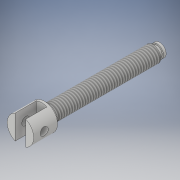
# Autodesk Inventor part: крепёж
Saved by Autodesk Inventor 2019 (Build 230136000, 136)
## iProperties
Created: 2019-04-29
Part Number: крепёж
Material: Типовые
Document SubType Name: Modeling
Designer: BarmanKaktus
Density: 1 g/cm^3
Appearance: По умолчанию
Author: BarmanKaktus
Autodesk Inventor part; units mm, degrees
sketch "Эскиз1" plane through (0, 0, 0) normal (0, 0, 1) x (1, 0, 0)
  circle A0 centre (0, 0) radius 3
  dimension "d0" = 6
  constraints: 1 centre point, 1 coincident
  measures "d0" diameter of A0
extrude "Выдавливание1" add sketch "Эскиз1" along normal blind 40
ref_plane "РабПлоскость1" through (0, 0, 40) normal (0, 0, 1) x (1, 0, 0)
sketch "Эскиз2" plane through (0, 0, 40) normal (0, 0, 1) x (1, 0, 0)
  circle A0 centre (0, 0) radius 5
  dimension "d4" = 10
  constraints: 1 centre point, 1 coincident
  measures "d4" diameter of A0
extrude "Выдавливание2" add sketch "Эскиз2" along normal blind 10
ref_plane "РабПлоскость2" through (0, 0, 50) normal (0, 0, 1) x (1, 0, 0)
sketch "Эскиз3" plane through (0, 0, 50) normal (0, 0, 1) x (1, 0, 0)
  line L0 (-2, 8) -> (2, 8)
  line L1 (2, 8) -> (2, -7)
  line L2 (2, -7) -> (-2, -7)
  line L3 (-2, -7) -> (-2, 8)
  point P0 (0, 0)
  dimension "d8" = 4
  dimension "d9" = 15
  constraints: 8 end point, 2 parallel, 1 horizontal, 1 perpendicular
  measures "d8" distance of L0.start L0.end
  measures "d9" distance of L0.end L1.end
extrude "Выдавливание3" cut sketch "Эскиз3" against normal blind 8
ref_plane "РабПлоскость3" through (-5, 0, 40) normal (1, 0, 0) x (0, 1, 0)
sketch "Эскиз4" plane through (-5, 0, 40) normal (1, 0, 0) x (0, 1, 0)
  circle A0 centre (0, 6) radius 1.5
  line L0 (4.5826, 10) -> (-4.5826, 10) projected
  point P0 (0, -40)
  dimension "d12" = 3
  dimension "d13" = 4
  constraints: 1 centre point
  measures "d12" diameter of A0
  measures "d13" distance from line of L0 A0.centre
extrude "Выдавливание4" cut sketch "Эскиз4" along normal blind 10
ref_plane "РабПлоскость4" through (0, 0, 0) normal (0, 0, -1) x (-1, 0, 0)
sketch "Эскиз5" plane through (0, 0, 0) normal (0, 0, -1) x (-1, 0, 0)
  circle A0 centre (0, 0) radius 2
  dimension "d17" = 4
  constraints: 1 centre point, 1 coincident
  measures "d17" diameter of A0
extrude "Выдавливание5" add sketch "Эскиз5" along normal blind 1.5
ref_plane "РабПлоскость5" through (0, 0, -1.5) normal (0, 0, -1) x (-1, 0, 0)
sketch "Эскиз6" plane through (0, 0, -1.5) normal (0, 0, -1) x (-1, 0, 0)
  circle A0 centre (0, 0) radius 2.5
  dimension "d21" = 5
  constraints: 1 centre point, 1 coincident
  measures "d21" diameter of A0
extrude "Выдавливание6" add sketch "Эскиз6" along normal blind 1
chamfer "Фаска1" distance 1 angle 45 1 edges at (-5, 0, 40)
thread "Резьба1" size "M6x1" class "6g" standard "ANSI Metric M Profile" full length
